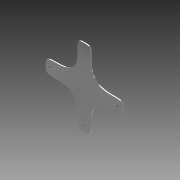
# Autodesk Inventor part: TopPlate
Saved by Autodesk Inventor 2011 SP1 (Build 150282100, 282)
## iProperties
Created: 2011-08-02
Part Number: TopPlate
Document SubType Name: Modeling
Designer: Nathan
Density: 1 g/cm^3
Author: Nathan
Autodesk Inventor part; units mm, degrees
ref_plane "YZ Plane" through (0, 0, 0) normal (1, 0, 0) x (0, 1, 0)
ref_plane "XZ Plane" through (0, 0, 0) normal (0, 1, 0) x (-1, 0, 0)
ref_plane "XY Plane" through (0, 0, 0) normal (0, 0, 1) x (1, 0, 0)
sketch "Sketch1" plane through (0, 0, 0) normal (0, 0, 1) x (1, 0, 0)
  spline S0 degree 5 poles (-63.5, 0) (-63.4959, -4.0863) (-63.3246, -10.8685) (-62.6474, -15.6962) (6.7202, 4.2103) (-21.6642, -81.0755) (0.2333, -51.0027) (21.59, -81.6082) (-6.041, 6.0357) (81.758, -21.457) (51.0727, -0.086) (81.7701, 21.7984) (-6.0259, -6.0316) (21.593, 81.7641) (0.2276, 51.0997) (-21.6558, 81.2362) (6.6904, -4.281) (-62.7361, 16.0116) (-63.3457, 10.9508) (-63.5041, 4.0947) (-63.5, 0) knots 0 0 0 0 0 0 0.074877 0.124852 0.182702 0.249872 0.317042 0.374892 0.432737 0.499846 0.566955 0.624801 0.682702 0.749872 0.817042 0.874943 0.924969 1 1 1 1 1 1
  line L0 (0, -6.1276) -> (0, 6.2502)
  line L1 (-5.7299, 0.0613) -> (8.1185, 0.0613)
  line L2 (0, 0) -> (10.1713, 10.1713)
  line L3 (0, 0) -> (14.3844, 0) construction
  point P0 (-18.941, -18.8184)
  point P1 (-9.1276, -61.7086)
  point P2 (0, -63.4387)
  point P3 (9.1276, -61.7086)
  point P4 (18.941, -18.8184)
  point P5 (61.8311, -9.005)
  point P6 (63.5, 0)
  point P7 (61.8311, 9.1276)
  point P8 (18.941, 18.941)
  point P9 (9.1276, 61.8311)
  point P10 (0, 63.5613)
  point P11 (-9.1276, 61.8311)
  point P12 (-18.941, 18.941)
  point P13 (-61.8311, 9.1276)
  point P14 (0, 55.9413)
  point P15 (55.9413, 0)
  point P16 (0, -55.8187)
  point P17 (-55.9413, 0)
  dimension "d0" = 127
  dimension "d1" = 127
  dimension "d2" = 45
  dimension "d14" = 55.88
  constraints: 18 symmetric about line, 8 end point, 2 horizontal, 2 vertical, 1 equal length, 1 perpendicular, 1 point on line, 16 other
  measures "d0" distance of point (-63.5, 0) point (63.5, 0)
  measures "d1" distance of point (0, -63.439) point (0, 63.561)
  measures "d2" angle of L3 L2
  measures "d14" distance from line of L1 point (0, 55.941)
extrude "Extrusion1" add sketch "Sketch1" against normal blind 1.5875 contours S0 | L0 L1 L2
hole "Hole1" at (0, 55.9413, 0) at (55.9413, 0, 0) at (0, -55.8187, 0) at (-55.9413, 0, 0) direction (0, 0, -1) diameter 3.302 end through all thread size "8-32 UNC" class "2B" standard "ANSI Unified Screw Threads"
equation "\"d1\" = d0"
body "Solid1"
